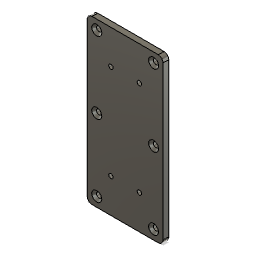
Jkk_to_2080_adapter v1 (Autodesk Fusion 360 design; units mm, degrees)
Autodesk Fusion 360 part; units mm, degrees
sketch "Skizze2" plane through (0, 0, 0) normal (0, 0, 1) x (1, 0, 0)
  line L0 (15, 50) -> (-15, 50)
  line L1 (-15, 50) -> (-15, -50)
  line L2 (-15, -50) -> (15, -50)
  line L3 (15, -50) -> (15, 50)
  line L4 (15, 50) -> (-15, -50) construction
  line L5 (-15, 50) -> (15, -50) construction
  circle A0 centre (15, 50) radius 2.3
  circle A1 centre (-15, 50) radius 2.3
  circle A2 centre (-15, -50) radius 2.3
  circle A3 centre (15, -50) radius 2.3
  line L6 (40, 86) -> (-40, 86)
  line L7 (-40, 86) -> (-40, -86)
  line L8 (-40, -86) -> (40, -86)
  line L9 (40, -86) -> (40, 86)
  line L10 (40, 86) -> (-40, -86) construction
  line L11 (-40, 86) -> (40, -86) construction
  line L12 (-30, -86) -> (-30, 86)
  line L13 (30, 86) -> (30, -86)
  line L14 (0, 0) -> (0, -50)
  circle A4 centre (-30, -76) radius 2.75
  circle A5 centre (-30, 0) radius 2.75
  circle A6 centre (-30, 76) radius 2.75
  line L15 (-30, 76) -> (30, 76)
  line L16 (-30, 0) -> (30, 0)
  line L17 (-30, -76) -> (30, -76)
  circle A7 centre (30, -76) radius 2.75
  circle A8 centre (30, 0) radius 2.75
  circle A9 centre (30, 76) radius 2.75
  dimension "d1" = 4.6
  dimension "d2" = 30
  dimension "d3" = 100
  dimension "d4" = 36
  dimension "d5" = 80
  dimension "d6" = 60
  dimension "d7" = 10
  dimension "d8" = 10
  dimension "d9" = 5.5
  constraint horizontal L0
  constraint perpendicular L0 L1
  constraint parallel L0 L2
  constraint parallel L1 L3
  constraint coincident L4 L14.start
  constraint coincident L5 L14.start
  constraint coincident L14.start origin
  constraint coincident L0.start L3.end
  constraint coincident L0.end L1.start
  constraint coincident L1.end L2.start
  constraint coincident L2.end L3.start
  constraint equal A0 A1
  constraint equal A0 A3
  constraint equal A2 A3
  constraint horizontal L6
  constraint perpendicular L6 L7
  constraint parallel L6 L8
  constraint parallel L7 L9
  constraint coincident L10 L14.start
  constraint coincident L11 L14.start
  constraint coincident L8 L12.start
  constraint coincident L6 L12.end
  constraint perpendicular L6 L12
  constraint coincident L6 L13.start
  constraint perpendicular L6 L13
  constraint midpoint L2 L14.end
  constraint symmetric L12 L13 L14
  constraint coincident L12 A4.centre
  constraint coincident L12 A5.centre
  constraint coincident L12 A6.centre
  constraint coincident A6.centre L15.start
  constraint coincident L13 L15.end
  constraint perpendicular L13 L15
  constraint coincident A5.centre L16.start
  constraint coincident L13 L16.end
  constraint perpendicular L13 L16
  constraint coincident A4.centre L17.start
  constraint coincident L13 L17.end
  constraint perpendicular L13 L17
  constraint coincident L17.end A7.centre
  constraint coincident L16.end A8.centre
  constraint coincident L15.end A9.centre
  constraint symmetric L6 L8 L16
  constraint equal A6 A9
  constraint equal A8 A9
  constraint equal A5 A8
  constraint equal A4 A5
  constraint equal A4 A7
  measures "d1" diameter of A0
  measures "d2" distance of L0.start L0.end
  measures "d3" distance of L0.start L2.end
  measures "d4" distance of L2.end L8
  measures "d5" distance of L7.end L8.end
  measures "d6" distance of L12 L13
  measures "d7" distance of L8 L17.end
  measures "d8" distance of L6 L15.end
  measures "d9" diameter of A8
extrude "Extrusion1" add sketch "Skizze2" against normal blind 6 contours L0 L1 L3 A0 A1 L12 L13 A5 A6 L15 L16 A8 A9 | L0 L1 L3 A0 A1 L16 | L1 L2 A2 L14 L16 | L1 L2 L3 A2 A3 L12 L13 A4 A5 L16 L17 A7 A8 | L2 L3 A3 L14 L16 | L6 L7 L8 L12 A4 A5 A6 | L6 L8 L9 L13 A7 A8 A9 | L6 L12 L13 A6 L15 A9 | L8 L12 L13 A4 L17 A7
fillet "Abrundung1" radius 5 4 edges at (40, -86, -3) (-40, -86, -3) (40, 86, -3) (-40, 86, -3)
hole "Bohrung1" at (30, 0, 0) at (30, 76, 0) at (30, -76, 0) at (-30, -76, 0) at (-30, 0, 0) at (-30, 76, 0) direction (0, 0, -1) diameter 5 depth 30 tip angle 118 countersink diameter 10.5 countersink angle 90
equation "d8 = d7"
